Autodesk Inventor part; units mm, degrees
(part 3 of 3)
  line L616 (61.1181, -65.6739) -> (61.0426, -65.6995) projected
  line L617 (61.0426, -65.6995) -> (60.9688, -65.7286) projected
  line L618 (60.9688, -65.7286) -> (60.8968, -65.7612) projected
  line L619 (60.8968, -65.7612) -> (60.8268, -65.7971) projected
  line L620 (60.8268, -65.7971) -> (60.7587, -65.8363) projected
  line L621 (60.7587, -65.8363) -> (60.6928, -65.8786) projected
  line L622 (60.6928, -65.8786) -> (60.6291, -65.9239) projected
  line L623 (60.6291, -65.9239) -> (60.5678, -65.9722) projected
  line L624 (60.5678, -65.9722) -> (60.5088, -66.0233) projected
  line L625 (60.5088, -66.0233) -> (60.4524, -66.0771) projected
  line L626 (60.4524, -66.0771) -> (60.3987, -66.1336) projected
  line L627 (60.3987, -66.1336) -> (60.3476, -66.1926) projected
  line L628 (60.3476, -66.1926) -> (60.2994, -66.254) projected
  line L629 (60.2994, -66.254) -> (60.2541, -66.3177) projected
  line L630 (60.2541, -66.3177) -> (60.2119, -66.3837) projected
  line L631 (60.2119, -66.3837) -> (60.1728, -66.4517) projected
  line L632 (60.1728, -66.4517) -> (60.1369, -66.5218) projected
  line L633 (60.1369, -66.5218) -> (60.1044, -66.5938) projected
  line L634 (60.1044, -66.5938) -> (60.0754, -66.6676) projected
  line L635 (60.0754, -66.6676) -> (60.0498, -66.7431) projected
  line L636 (60.0498, -66.7431) -> (60.028, -66.8202) projected
  line L637 (60.028, -66.8202) -> (60.0099, -66.8989) projected
  line L638 (60.0099, -66.8989) -> (59.9956, -66.9789) projected
  line L639 (59.9956, -66.9789) -> (59.9853, -67.0602) projected
  point P0 (0, 0)
extrude "Extrusion3" add sketch "Sketch5" along normal blind 4
sketch "Sketch6" plane through (0, 0, 4) normal (0, 0, 1) x (1, 0, 0)
  line L0 (73.6013, -59.9669) -> (73.6037, -63.2169) projected
  arc A0 (59.1805, -48.8249) -> (48.8055, -59.2842) centre (61.5989, -61.5991) ccw projected
  circle A1 centre (61.5989, -61.5991) radius 8.75
  circle A2 centre (61.5989, -56.8491) radius 3.15
  line L1 (63.1737, -59.5772) -> (64.1374, -61.2465)
  line L2 (62.5622, -63.977) -> (60.6391, -63.9784)
  circle A3 centre (57.4891, -63.9808) radius 3.15
  circle A4 centre (65.7122, -63.9746) radius 3.15
  arc A5 (66.294, -60.8788) -> (64.5707, -57.8936) centre (61.5989, -61.5991) ccw
  arc A6 (58.6271, -57.8936) -> (56.9028, -60.8858) centre (61.5989, -61.5991) ccw
  arc A7 (59.8829, -66.0283) -> (63.3215, -66.0257) centre (61.5989, -61.5991) ccw
  point P0 (0, 0)
  dimension "d25" = 4.75
  constraints: 16 point on circle, 7 centre point, 4 end point, 2 coincident, 1 perpendicular
  measures "d25" radius of A6
extrude "Extrusion4" cut sketch "Sketch6" against normal blind 2 contours A2 | A3 | A4
sketch "Sketch7" plane through (57.4891, -63.9808, 2) normal (0, 0, 1) x (1, 0, 0)
  circle A0 centre (0, 0) radius 3.15 projected
  circle A1 centre (4.1098, 7.1317) radius 3.15 projected
  circle A2 centre (8.2231, 0.0061) radius 3.15 projected
  circle A3 centre (0, 0) radius 3.5
  circle A4 centre (4.1098, 7.1317) radius 3.5
  circle A5 centre (8.2231, 0.0061) radius 3.5
  point P0 (-57.4891, 63.9808)
  dimension "d19" = 7
  dimension "d20" = 7
  dimension "d21" = 7
  constraints: 3 centre point, 3 coincident
  measures "d19" diameter of A3
  measures "d20" diameter of A4
  measures "d21" diameter of A5
extrude "Extrusion5" cut sketch "Sketch7" against normal blind 2.5 contours A0 | A1 | A2 | A3 | A4 | A5
fillet "Fillet1" radius 0.4 6 edges at (58.0989, -56.8491, 2) (64.5707, -55.8046, 4) (53.9891, -63.9808, 2) (55.0954, -61.9332, 4) (65.1305, -67.0704, 2) (65.1305, -67.0704, 4)
sketch "Sketch10" plane through (0, 0, 0) normal (0, 0, -1) x (-1, 0, 0)
  line L0 (-59.975, -49.595) -> (-59.975, -52.845) projected
  line L1 (-59.975, -52.845) -> (-63.225, -52.845) projected
  line L2 (-63.225, -52.845) -> (-63.225, -49.595) projected
  line L3 (-63.225, -49.595) -> (-59.975, -49.595) projected
  line L4 (-52.8934, -63.4537) -> (-49.8915, -64.6991) projected
  line L5 (-49.8915, -64.6991) -> (-51.1369, -67.701) projected
  line L6 (-51.1369, -67.701) -> (-54.1388, -66.4556) projected
  line L7 (-54.1388, -66.4556) -> (-52.8934, -63.4537) projected
  line L8 (-54.2646, -66.6445) -> (-51.9695, -68.9456) projected
  line L9 (-51.9695, -68.9456) -> (-54.2706, -71.2407) projected
  line L10 (-54.2706, -71.2407) -> (-56.5657, -68.9397) projected
  line L11 (-56.5657, -68.9397) -> (-54.2646, -66.6445) projected
  line L12 (-56.7527, -69.0659) -> (-55.5107, -72.0693) projected
  line L13 (-55.5107, -72.0693) -> (-58.514, -73.3112) projected
  line L14 (-58.514, -73.3112) -> (-59.756, -70.3079) projected
  line L15 (-59.756, -70.3079) -> (-56.7527, -69.0659) projected
  line L16 (-59.9793, -70.3529) -> (-59.9813, -73.6029) projected
  line L17 (-59.9813, -73.6029) -> (-63.2313, -73.6008) projected
  line L18 (-63.2313, -73.6008) -> (-63.2293, -70.3508) projected
  line L19 (-63.2293, -70.3508) -> (-59.9793, -70.3529) projected
  line L20 (-63.4534, -70.3067) -> (-64.6994, -73.3084) projected
  line L21 (-64.6994, -73.3084) -> (-67.7011, -72.0624) projected
  line L22 (-67.7011, -72.0624) -> (-66.455, -69.0607) projected
  line L23 (-66.455, -69.0607) -> (-63.4534, -70.3067) projected
  line L24 (-66.6438, -68.9351) -> (-68.9435, -71.2317) projected
  line L25 (-68.9435, -71.2317) -> (-71.24, -68.932) projected
  line L26 (-71.24, -68.932) -> (-68.9403, -66.6355) projected
  line L27 (-68.9403, -66.6355) -> (-66.6438, -68.9351) projected
  line L28 (-69.0665, -66.4474) -> (-72.0699, -67.6893) projected
  line L29 (-72.0699, -67.6893) -> (-73.3118, -64.686) projected
  line L30 (-73.3118, -64.686) -> (-70.3085, -63.4441) projected
  line L31 (-70.3085, -63.4441) -> (-69.0665, -66.4474) projected
  line L32 (-70.3079, -59.7483) -> (-73.3095, -58.5022) projected
  line L33 (-73.3095, -58.5022) -> (-72.0634, -55.5006) projected
  line L34 (-72.0634, -55.5006) -> (-69.0618, -56.7467) projected
  line L35 (-69.0618, -56.7467) -> (-70.3079, -59.7483) projected
  line L36 (-68.9355, -56.5569) -> (-71.2319, -54.2571) projected
  line L37 (-71.2319, -54.2571) -> (-68.932, -51.9607) projected
  line L38 (-68.932, -51.9607) -> (-66.6357, -54.2606) projected
  line L39 (-66.6357, -54.2606) -> (-68.9355, -56.5569) projected
  line L40 (-66.4458, -54.1331) -> (-67.6871, -51.1295) projected
  line L41 (-67.6871, -51.1295) -> (-64.6835, -49.8882) projected
  line L42 (-64.6835, -49.8882) -> (-63.4422, -52.8918) projected
  line L43 (-63.4422, -52.8918) -> (-66.4458, -54.1331) projected
  line L44 (-59.7474, -52.8928) -> (-58.5019, -49.891) projected
  line L45 (-58.5019, -49.891) -> (-55.5, -51.1366) projected
  line L46 (-55.5, -51.1366) -> (-56.7456, -54.1384) projected
  line L47 (-56.7456, -54.1384) -> (-59.7474, -52.8928) projected
  line L48 (-56.5557, -54.2647) -> (-54.2559, -51.9683) projected
  line L49 (-54.2559, -51.9683) -> (-51.9595, -54.2681) projected
  line L50 (-51.9595, -54.2681) -> (-54.2593, -56.5645) projected
  line L51 (-54.2593, -56.5645) -> (-56.5557, -54.2647) projected
  line L52 (-54.1334, -56.752) -> (-51.1301, -55.5101) projected
  line L53 (-51.1301, -55.5101) -> (-49.8882, -58.5135) projected
  line L54 (-49.8882, -58.5135) -> (-52.8916, -59.7554) projected
  line L55 (-52.8916, -59.7554) -> (-54.1334, -56.752) projected
  arc A0 (-52.9038, -71.2653) -> (-48.6, -61.6029) centre (-61.5843, -61.6091) ccw projected
  arc A1 (-48.6, -61.6029) -> (-48.8055, -59.2842) centre (-61.5557, -61.583) ccw projected
  arc A2 (-48.8055, -59.2842) -> (-59.1805, -48.8249) centre (-61.5989, -61.5991) ccw projected
  arc A3 (-59.1805, -48.8249) -> (-74.163, -58.2471) centre (-61.5986, -61.6031) ccw projected
  arc A4 (-74.163, -58.2471) -> (-72.8082, -68.1903) centre (-61.5989, -61.5991) ccw projected
  arc A5 (-72.8082, -68.1903) -> (-52.9038, -71.2653) centre (-61.6004, -61.5999) ccw projected
  circle A6 centre (-61.5989, -56.8491) radius 3.5 projected
  circle A7 centre (-65.7122, -63.9746) radius 3.5 projected
  circle A8 centre (-57.4891, -63.9808) radius 3.5 projected
  line L56 (-59.975, -49.595) -> (-59.975, -52.845) projected
  line L57 (-59.975, -52.845) -> (-63.225, -52.845) projected
  line L58 (-63.225, -52.845) -> (-63.225, -49.595) projected
  line L59 (-63.225, -49.595) -> (-59.975, -49.595) projected
  line L60 (-52.8934, -63.4537) -> (-49.8915, -64.6991) projected
  line L61 (-49.8915, -64.6991) -> (-51.1369, -67.701) projected
  line L62 (-51.1369, -67.701) -> (-54.1388, -66.4556) projected
  line L63 (-54.1388, -66.4556) -> (-52.8934, -63.4537) projected
  line L64 (-54.2646, -66.6445) -> (-51.9695, -68.9456) projected
  line L65 (-51.9695, -68.9456) -> (-54.2706, -71.2407) projected
  line L66 (-54.2706, -71.2407) -> (-56.5657, -68.9397) projected
  line L67 (-56.5657, -68.9397) -> (-54.2646, -66.6445) projected
  line L68 (-56.7527, -69.0659) -> (-55.5107, -72.0693) projected
  line L69 (-55.5107, -72.0693) -> (-58.514, -73.3112) projected
  line L70 (-58.514, -73.3112) -> (-59.756, -70.3079) projected
  line L71 (-59.756, -70.3079) -> (-56.7527, -69.0659) projected
  line L72 (-59.9793, -70.3529) -> (-59.9813, -73.6029) projected
  line L73 (-59.9813, -73.6029) -> (-63.2313, -73.6008) projected
  line L74 (-63.2313, -73.6008) -> (-63.2293, -70.3508) projected
  line L75 (-63.2293, -70.3508) -> (-59.9793, -70.3529) projected
  line L76 (-63.4534, -70.3067) -> (-64.6994, -73.3084) projected
  line L77 (-64.6994, -73.3084) -> (-67.7011, -72.0624) projected
  line L78 (-67.7011, -72.0624) -> (-66.455, -69.0607) projected
  line L79 (-66.455, -69.0607) -> (-63.4534, -70.3067) projected
  line L80 (-66.6438, -68.9351) -> (-68.9435, -71.2317) projected
  line L81 (-68.9435, -71.2317) -> (-71.24, -68.932) projected
  line L82 (-71.24, -68.932) -> (-68.9403, -66.6355) projected
  line L83 (-68.9403, -66.6355) -> (-66.6438, -68.9351) projected
  line L84 (-69.0665, -66.4474) -> (-72.0699, -67.6893) projected
  line L85 (-72.0699, -67.6893) -> (-73.3118, -64.686) projected
  line L86 (-73.3118, -64.686) -> (-70.3085, -63.4441) projected
  line L87 (-70.3085, -63.4441) -> (-69.0665, -66.4474) projected
  line L88 (-70.3079, -59.7483) -> (-73.3095, -58.5022) projected
  line L89 (-73.3095, -58.5022) -> (-72.0634, -55.5006) projected
  line L90 (-72.0634, -55.5006) -> (-69.0618, -56.7467) projected
  line L91 (-69.0618, -56.7467) -> (-70.3079, -59.7483) projected
  line L92 (-68.9355, -56.5569) -> (-71.2319, -54.2571) projected
  line L93 (-71.2319, -54.2571) -> (-68.932, -51.9607) projected
  line L94 (-68.932, -51.9607) -> (-66.6357, -54.2606) projected
  line L95 (-66.6357, -54.2606) -> (-68.9355, -56.5569) projected
  line L96 (-66.4458, -54.1331) -> (-67.6871, -51.1295) projected
  line L97 (-67.6871, -51.1295) -> (-64.6835, -49.8882) projected
  line L98 (-64.6835, -49.8882) -> (-63.4422, -52.8918) projected
  line L99 (-63.4422, -52.8918) -> (-66.4458, -54.1331) projected
  line L100 (-59.7474, -52.8928) -> (-58.5019, -49.891) projected
  line L101 (-58.5019, -49.891) -> (-55.5, -51.1366) projected
  line L102 (-55.5, -51.1366) -> (-56.7456, -54.1384) projected
  line L103 (-56.7456, -54.1384) -> (-59.7474, -52.8928) projected
  line L104 (-56.5557, -54.2647) -> (-54.2559, -51.9683) projected
  line L105 (-54.2559, -51.9683) -> (-51.9595, -54.2681) projected
  line L106 (-51.9595, -54.2681) -> (-54.2593, -56.5645) projected
  line L107 (-54.2593, -56.5645) -> (-56.5557, -54.2647) projected
  line L108 (-54.1334, -56.752) -> (-51.1301, -55.5101) projected
  line L109 (-51.1301, -55.5101) -> (-49.8882, -58.5135) projected
  line L110 (-49.8882, -58.5135) -> (-52.8916, -59.7554) projected
  line L111 (-52.8916, -59.7554) -> (-54.1334, -56.752) projected
  line L112 (-52.8505, -59.9795) -> (-49.6005, -59.9784) projected
  line L113 (-49.6005, -59.9784) -> (-49.5995, -63.2284) projected
  line L114 (-49.5995, -63.2284) -> (-52.8495, -63.2295) projected
  line L115 (-52.8495, -63.2295) -> (-52.8505, -59.9795) projected
  line L116 (-70.3537, -63.2194) -> (-73.6037, -63.2169) projected
  line L117 (-73.6037, -63.2169) -> (-73.6013, -59.9669) projected
  line L118 (-73.6013, -59.9669) -> (-70.3513, -59.9694) projected
  line L119 (-70.3513, -59.9694) -> (-70.3537, -63.2194) projected
  arc A9 (-52.9038, -71.2653) -> (-48.6, -61.6029) centre (-61.5843, -61.6091) ccw projected
  arc A10 (-48.6, -61.6029) -> (-48.8055, -59.2842) centre (-61.5557, -61.583) ccw projected
  arc A11 (-48.8055, -59.2842) -> (-59.1805, -48.8249) centre (-61.5989, -61.5991) ccw projected
  arc A12 (-59.1805, -48.8249) -> (-74.163, -58.2471) centre (-61.5986, -61.6031) ccw projected
  arc A13 (-74.163, -58.2471) -> (-72.8082, -68.1903) centre (-61.5989, -61.5991) ccw projected
  arc A14 (-72.8082, -68.1903) -> (-52.9038, -71.2653) centre (-61.6004, -61.5999) ccw projected
  point P0 (0, 0)
extrude "Extrusion7" add sketch "Sketch10" along normal blind 1 contours L0 L1 L2 L3 | L4 L5 L6 L7 | L8 L9 L10 L11 | L12 L13 L14 L15 | L16 L17 L18 L19 | L20 L21 L22 L23 | L24 L25 L26 L27 | L28 L29 L30 L31 | L32 L33 L34 L35 | L36 L37 L38 L39 | L40 L41 L42 L43 | L44 L45 L46 L47 | L48 L49 L50 L51 | L52 L53 L54 L55 | A5 A4 A3 A2 A1 A0 | A6 | A7 | A8 | L112 L113 L114 L115 | L116 L117 L118 L119
sketch "Sketch11" plane through (0, 0, 4) normal (0, 0, 1) x (1, 0, 0)
  arc A0 (52.9038, -71.2653) -> (72.8082, -68.1903) centre (61.6004, -61.5999) ccw projected
  arc A1 (48.6, -61.6029) -> (52.9038, -71.2653) centre (61.5843, -61.6091) ccw projected
  arc A2 (48.8055, -59.2842) -> (48.6, -61.6029) centre (61.5557, -61.583) ccw projected
  arc A3 (59.1805, -48.8249) -> (48.8055, -59.2842) centre (61.5989, -61.5991) ccw projected
  arc A4 (74.163, -58.2471) -> (59.1805, -48.8249) centre (61.5986, -61.6031) ccw projected
  arc A5 (72.8082, -68.1903) -> (74.163, -58.2471) centre (61.5989, -61.5991) ccw projected
  circle A6 centre (57.4891, -63.9808) radius 3.55 projected
  arc A7 (48.8055, -59.2842) -> (48.6, -61.6029) centre (61.5557, -61.583) ccw projected
  arc A8 (48.6, -61.6029) -> (52.9038, -71.2653) centre (61.5843, -61.6091) ccw projected
  arc A9 (52.9038, -71.2653) -> (72.8082, -68.1903) centre (61.6004, -61.5999) ccw projected
  arc A10 (72.8082, -68.1903) -> (74.163, -58.2471) centre (61.5989, -61.5991) ccw projected
  arc A11 (74.163, -58.2471) -> (59.1805, -48.8249) centre (61.5986, -61.6031) ccw projected
  arc A12 (59.1805, -48.8249) -> (48.8055, -59.2842) centre (61.5989, -61.5991) ccw projected
  line L0 (73.6037, -63.2169) -> (70.3537, -63.2194) projected
  line L1 (70.3537, -63.2194) -> (70.3513, -59.9694) projected
  line L2 (70.3513, -59.9694) -> (73.6013, -59.9669) projected
  line L3 (73.6013, -59.9669) -> (73.6037, -63.2169) projected
  line L4 (49.6005, -59.9784) -> (52.8505, -59.9795) projected
  line L5 (52.8505, -59.9795) -> (52.8495, -63.2295) projected
  line L6 (52.8495, -63.2295) -> (49.5995, -63.2284) projected
  line L7 (49.5995, -63.2284) -> (49.6005, -59.9784) projected
  line L8 (51.1301, -55.5101) -> (54.1334, -56.752) projected
  line L9 (54.1334, -56.752) -> (52.8916, -59.7554) projected
  line L10 (52.8916, -59.7554) -> (49.8882, -58.5135) projected
  line L11 (49.8882, -58.5135) -> (51.1301, -55.5101) projected
  line L12 (54.2559, -51.9683) -> (56.5557, -54.2647) projected
  line L13 (56.5557, -54.2647) -> (54.2593, -56.5645) projected
  line L14 (54.2593, -56.5645) -> (51.9595, -54.2681) projected
  line L15 (51.9595, -54.2681) -> (54.2559, -51.9683) projected
  line L16 (58.5019, -49.891) -> (59.7474, -52.8928) projected
  line L17 (59.7474, -52.8928) -> (56.7456, -54.1384) projected
  line L18 (56.7456, -54.1384) -> (55.5, -51.1366) projected
  line L19 (55.5, -51.1366) -> (58.5019, -49.891) projected
  line L20 (67.6871, -51.1295) -> (66.4458, -54.1331) projected
  line L21 (66.4458, -54.1331) -> (63.4422, -52.8918) projected
  line L22 (63.4422, -52.8918) -> (64.6835, -49.8882) projected
  line L23 (64.6835, -49.8882) -> (67.6871, -51.1295) projected
  line L24 (71.2319, -54.2571) -> (68.9355, -56.5569) projected
  line L25 (68.9355, -56.5569) -> (66.6357, -54.2606) projected
  line L26 (66.6357, -54.2606) -> (68.932, -51.9607) projected
  line L27 (68.932, -51.9607) -> (71.2319, -54.2571) projected
  line L28 (73.3095, -58.5022) -> (70.3079, -59.7483) projected
  line L29 (70.3079, -59.7483) -> (69.0618, -56.7467) projected
  line L30 (69.0618, -56.7467) -> (72.0634, -55.5006) projected
  line L31 (72.0634, -55.5006) -> (73.3095, -58.5022) projected
  line L32 (72.0699, -67.6893) -> (69.0665, -66.4474) projected
  line L33 (69.0665, -66.4474) -> (70.3085, -63.4441) projected
  line L34 (70.3085, -63.4441) -> (73.3118, -64.686) projected
  line L35 (73.3118, -64.686) -> (72.0699, -67.6893) projected
  line L36 (68.9435, -71.2317) -> (66.6438, -68.9351) projected
  line L37 (66.6438, -68.9351) -> (68.9403, -66.6355) projected
  line L38 (68.9403, -66.6355) -> (71.24, -68.932) projected
  line L39 (71.24, -68.932) -> (68.9435, -71.2317) projected
  line L40 (64.6994, -73.3084) -> (63.4534, -70.3067) projected
  line L41 (63.4534, -70.3067) -> (66.455, -69.0607) projected
  line L42 (66.455, -69.0607) -> (67.7011, -72.0624) projected
  line L43 (67.7011, -72.0624) -> (64.6994, -73.3084) projected
  line L44 (59.9813, -73.6029) -> (59.9793, -70.3529) projected
  line L45 (59.9793, -70.3529) -> (63.2293, -70.3508) projected
  line L46 (63.2293, -70.3508) -> (63.2313, -73.6008) projected
  line L47 (63.2313, -73.6008) -> (59.9813, -73.6029) projected
  line L48 (55.5107, -72.0693) -> (56.7527, -69.0659) projected
  line L49 (56.7527, -69.0659) -> (59.756, -70.3079) projected
  line L50 (59.756, -70.3079) -> (58.514, -73.3112) projected
  line L51 (58.514, -73.3112) -> (55.5107, -72.0693) projected
  line L52 (51.9695, -68.9456) -> (54.2646, -66.6445) projected
  line L53 (54.2646, -66.6445) -> (56.5657, -68.9397) projected
  line L54 (56.5657, -68.9397) -> (54.2706, -71.2407) projected
  line L55 (54.2706, -71.2407) -> (51.9695, -68.9456) projected
  line L56 (49.8915, -64.6991) -> (52.8934, -63.4537) projected
  line L57 (52.8934, -63.4537) -> (54.1388, -66.4556) projected
  line L58 (54.1388, -66.4556) -> (51.1369, -67.701) projected
  line L59 (51.1369, -67.701) -> (49.8915, -64.6991) projected
  line L60 (59.975, -52.845) -> (59.975, -49.595) projected
  line L61 (59.975, -49.595) -> (63.225, -49.595) projected
  line L62 (63.225, -49.595) -> (63.225, -52.845) projected
  line L63 (63.225, -52.845) -> (59.975, -52.845) projected
  circle A13 centre (61.5989, -56.8491) radius 3.55 projected
  circle A14 centre (65.7122, -63.9746) radius 3.55 projected
  circle A15 centre (61.6021, -61.5994) radius 0.9
  line L64 (61.6025, -63.2259) -> (61.6043, -70.3518)
  line L65 (52.85, -61.6045) -> (60.0416, -61.5135)
  line L66 (63.1555, -61.5118) -> (70.3525, -61.5944)
  circle A16 centre (57.4891, -63.9808) radius 3.55 projected
  line L67 (73.6037, -63.2169) -> (70.3537, -63.2194) projected
  circle A17 centre (61.5989, -56.8491) radius 3.55 projected
  circle A18 centre (65.7122, -63.9746) radius 3.55 projected
  line L68 (61.6, -52.845) -> (61.6002, -53.2991)
  point P0 (0, 0)
  dimension "d30" = 1.8
  constraints: 8 end point, 4 midpoint, 1 centre point, 1 point on line, 6 other
  measures "d30" diameter of A15
extrude "Extrusion8" cut sketch "Sketch11" against normal blind 3.5 contours A15
body "Solid1"
